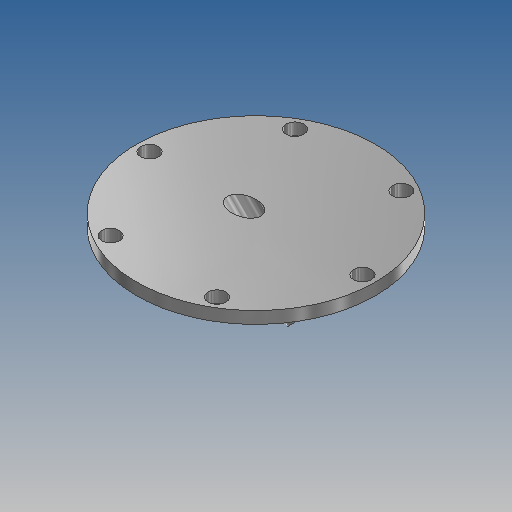
# Autodesk Inventor part: P021
Saved by Autodesk Inventor 2021.4 (Build 254397000, 397)
## iProperties
Created: 2022-06-06
Part Number: P021
Material: Aluminium
Document SubType Name: Modeling
Designer: Rémi Heredero
Density: 2.7 g/cm^3
Appearance: Aluminum - Dark
Author: Rémi Heredero
Title: Bouchon Carter Vilbrequin
Autodesk Inventor part; units mm, degrees
ref_plane "YZ Plane" through (0, 0, 0) normal (1, 0, 0) x (0, 1, 0)
ref_plane "XZ Plane" through (0, 0, 0) normal (0, 1, 0) x (-1, 0, 0)
ref_plane "XY Plane" through (0, 0, 0) normal (0, 0, 1) x (1, 0, 0)
sketch "Sketch2" plane through (0, 0, 0) normal (0, 0, 1) x (1, 0, 0)
  circle A0 centre (0, 0) radius 30
  dimension "d0" = 60
  constraints: 1 centre point, 1 coincident
  measures "d0" diameter of A0
extrude "Extrusion1" add sketch "Sketch2" along normal blind 3
sketch "Sketch5" plane through (0, 0, 0) normal (0, 0, -1) x (-1, 0, 0)
  circle A0 centre (26.75, 0) radius 1.621 construction
  circle A1 centre (0, 0) radius 23.5 construction
  line L0 (-36.5, 35) -> (38.5, 35) construction
  line L1 (-36.5, -35) -> (-36.5, 35) construction
  line L2 (38.5, -35) -> (-36.5, -35) construction
  line L3 (38.5, 35) -> (38.5, -35) construction
  circle A2 centre (13.375, 23.1662) radius 1.621 projected
  circle A3 centre (-26.75, 0) radius 1.621 projected
  circle A4 centre (13.375, -23.1662) radius 1.621 projected
  circle A5 centre (-13.375, -23.1662) radius 1.621 projected
  circle A6 centre (-13.375, 23.1662) radius 1.621 projected
  point P0 (-55.25, 0)
  point P1 (13.375, 23.1662)
  point P2 (-13.375, 23.1662)
  point P3 (-26.75, 0)
  point P4 (-13.375, -23.1662)
  point P5 (13.375, -23.1662)
  dimension "d26" = 360
  constraints: 1 coincident, 7 other
hole "Hole2" at (55.25, 0, 0) at (-13.375, -23.1662, 0) at (-26.75, 0, 0) at (-13.375, 23.1662, 0) at (13.375, 23.1662, 0) at (26.75, 0, 0) at (13.375, -23.1662, 0) direction (0, 0, 1) diameter 4.5 end through all start extended yes clearance for "Countersunk Flat Head Screw ISO 2009/7046" size "M4" standard "ISO"
sketch "Sketch7" plane through (0, 0, 0) normal (0, 1, 0) x (-1, 0, 0)
  line L0 (0, 0) -> (-31.8943, -31.8943)
  line L1 (-24.5, 0) -> (-29, 0) construction
  line L2 (15.625, 0) -> (11.125, 0) construction
  line L3 (15.625, 0) -> (11.125, 0) construction
  line L4 (29, 0) -> (24.5, 0) construction
  line L5 (-11.125, 0) -> (-15.625, 0) construction
  line L6 (-11.125, 0) -> (-15.625, 0) construction
  line L7 (30, 0) -> (-30, 0) construction
  line L8 (30, 0) -> (-30, 0) construction
  line L9 (8.7574, 13) -> (-14.9497, -10.7071)
  line L10 (-15.6569, -10) -> (7.3431, 13)
  line L11 (7.3431, 13) -> (8.7574, 13)
  line L12 (30, 3) -> (-30, 3) construction
  line L13 (30, 0) -> (-30, 0) construction
  line L14 (-15.6569, -10) -> (-14.9497, -10.7071)
  dimension "d28" = 6
  dimension "d29" = 1
  dimension "d31" = 45
  dimension "d33" = 10
  dimension "d34" = 10
  constraints: 12 end point, 2 parallel, 1 perpendicular, 1 other
  measures "d28" diameter of L9 L0
  measures "d29" distance of L9.end L10.start
  measures "d31" angle to the sketch x axis of L0
  measures "d33" distance from line of L7 L10.start
  measures "d34" distance between parallel lines of L11 L12
revolve "Revolution1" add sketch "Sketch7" angle 360 about axis through (0, 0, 0) along (0.7071068, 0, -0.7071068)
sketch "Sketch8" plane through (12.8284, 0, -12.8284) normal (0.7071068, 0, -0.7071068) x (-0.7071068, 0, -0.7071068)
  circle A0 centre (0, 0) radius 3 projected
  circle A1 centre (0, 0) radius 4 construction
  point P0 (0, 0)
extrude "Extrusion2" cut sketch "Sketch8" against normal through all
sketch "Sketch9" plane through (0, 0, 3) normal (0, 0, 1) x (1, 0, 0)
  ellipse E0 centre (-3, 0) end of major axis (2.6569, 0) minor radius 4 projected
  circle A0 centre (26.75, 0) radius 2.25 projected
  circle A1 centre (-13.375, 23.1662) radius 2.25 projected
  circle A2 centre (-13.375, -23.1662) radius 2.25 projected
  circle A3 centre (-26.75, 0) radius 2.25 projected
  circle A4 centre (13.375, 23.1662) radius 2.25 projected
  circle A5 centre (13.375, -23.1662) radius 2.25 projected
  circle A6 centre (0, 0) radius 30 projected
extrude "Extrusion3" cut sketch "Sketch9" along normal through all contours E0 | A6
thread "Thread1" size "M6x1" class "6H" standard "ISO Metric profile" length 10
chamfer "Chamfer1" distance 0.5 angle 45 2 edges at (12.8284, -3, -12.8284) (12.8284, 3, -12.8284)
body "Solid1"
